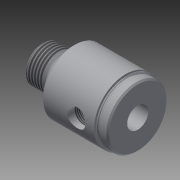
# Autodesk Inventor part: 12R000-0_rod_guide
Saved by Autodesk Inventor 2014 SP2 (Build 180246200, 246)
## iProperties
Created: 2019-01-29
Part Number: 12R000-0_rod_guide
Material: Generic
Catalog Web Link: www.cadenas.de
Description: Rod Guide-Original Line - Standard Air Cylinders
Vendor: BIMBA
Document SubType Name: Modeling
Designer: psadmin
Manufacturer: BIMBA
Mass: 28.8559 g
Surface Area: 85.2183 cm^2
Volume: 28.8559 cm^3
Density: 1 g/cm^3
Appearance: PSOLRGB-211-211-211
Category: PARTsolutions
Company: BIMBA
Title: 12R000-0_rod_guide
Author: Cadenas PARTsolutions
Comments: Original Line - Standard Air Cylinders
PSOL_IDENT_0: {$CADENAS_DATA\23d-libs\bimba\bimba\bimba_imperial\bimba_full_line\original_line_cylinders\standard_
PSOL_IDENT_1: air_cylinders\rod_guide.prj},251 {VTYP=3D},{NB=12R000-0_rod_guide},{LINA=12R000-0_rod_guide},{NN=Rod
PSOL_IDENT_2: Guide},{DATE=21.03.2018 14:31:21},{GEOMDATE=09.11.2017 12:44:00},{VERSION=},{LINEID=70},{WBVAR=MNT,
PSOL_IDENT_3: ACTING,NR,K,Q,T1,T2,T3,T4,MB,TRIM,CUSH,RODTRANS},{WBNUMERIC=MB,TRIM,CUSH,RODTRANS}  {NB=12R000-0_rod
PSOL_IDENT_4: _guide},{LINA=12R000-0_rod_guide},{KT=DUMMY},{PN=12R000},{BORE=1.25000000},{BOREPN=12},{MNT=},{MNTAL
PSOL_IDENT_5: G='' , 'Front Nose'},{ACTING=R},{ACTINGALG= '' , 'Single Acting' , 'R' , 'Reverse/Double Acting' },{
PSOL_IDENT_6: NR=},{NRALG= '' , 'N/A' },{K=},{Q=},{QALG= '' , 'Without Side Ported Rear Head' , 'Q' , 'With Side P
PSOL_IDENT_7: orted Rear Head' },{T1=},{T2=},{T3=},{T4=},{MB=0},{A1=2.0000},{A1N=1.5620},{A1P=2.0000},{A1B=0.0000}
PSOL_IDENT_8: ,{A2=0.6240},{A2N=0.6240},{A2P=0.6240},{A3=1.1250},{A3N=0.3110},{A3P=1.1250},{A4=0.2525},{A4N=0.6280
PSOL_IDENT_9: },{A4P=0.2525},{A5=0.0400},{A6=0.0000},{A6N=0.3750},{A6P=0.0000},{A7=0.4000},{A7N=0.9140},{A7P=0.400
PSOL_IDENT_10: 0},{A8=0.0300},{A8N=0.0300},{A8NR=0.0300},{D1=1.3265},{D1N=1.3265},{D1P=1.3265},{D1B=0.0000},{D2=1.2
PSOL_IDENT_11: 615},{D3=0.0000},{D3N=0.8120},{D3P=0.0000},{D4=0.8750},{D4N=0.4730},{D4P=0.8750},{D4NR=0.4395},{D5=0
PSOL_IDENT_12: .4420},{D5N=0.4420},{D5NR=0.4395},{C1=0.060},{C2=0.0300},{C2N=0.0600},{C2P=0.0300},{C3=0.0000},{C3N=
PSOL_IDENT_13: 0.0000},{C3P=0.0000},{C4=0.0600},{C4N=0.0600},{C4P=0.0600},{NDM=0.7500},{NDMN=0.7500},{NDMP=0.7500},
PSOL_IDENT_14: {TAB=UNF},{D6=0.7475},{D6N=0.7475},{D6P=0.7475},{A9=0.0940},{A9N=0.0940},{A9P=0.0940},{D7=0.6535},{D
PSOL_IDENT_15: 7N=0.6535},{D7P=0.6535},{A10=0.0965},{A10N=0.0965},{A10P=0.0965},{R1=0.0400},{R1N=0.0400},{R1P=0.040
PSOL_IDENT_16: 0},{D8=0.8750},{D9=0.7500},{D10=0.6880},{A11=0.9490},{A12=1.0740},{A13=1.2400},{A14=0.6250},{A14N=0.
PSOL_IDENT_17: 6250},{A14B=0.0000},{D11=0.2500},{D11N=0.2500},{NDM2=0.4050},{NDM2N=0.4050},{NDM2DP=0.3750},{THREAD=
PSOL_IDENT_18: 0},{HEX=0.4375},{HEXN=0.4375},{S1=0.0000},{B1=0.0000},{B2=0.0000},{B22=0.0000},{DB=0.0000},{B3=0.000
PSOL_IDENT_19: 0},{B4=0.0000},{X1=0.0000},{X2=0.0000},{NDM3=0.0000},{NDM4=0.0000},{NDM4DP=0.0000},{DD=0.0000},{CB=0
PSOL_IDENT_20: .0000},{CBDP=0.0000},{PORT=1},{XT=0.0000},{XTX=0.0000},{XT1=0.0000},{XT2=0.0000},{NDMH=0.0000},{OD=1
PSOL_IDENT_21: .3265},{ID=1.2615},{G=0.0000},{PNUT=0.5300},{TRIM=0},{C11=0.0000},{C22=0.0000},{C33=0.0000},{C44=0.0
PSOL_IDENT_22: 000},{C55=0.0000},{CD1=0.0000},{CD2=0.0000},{CD3=0.0000},{CNDM3=0.0000},{CTAB3=0.0000},{CUSH=0},{XX=
PSOL_IDENT_23: 0.00000},{LCD=0.0000},{RODTRANS=0.00000}
NN: Rod Guide
NT: Original Line - Standard Air Cylinders
NB: 12R000-0_rod_guide
NBSYN: $PN.-$RODTRANS._rod_guide
LINA: 12R000-0_rod_guide
BORE: 0
BOREPN: 12
MNT: Front Nose
MNTALG: '' , 'Front Nose'
ACTING: Reverse/Double Acting
NR: N/A
K: Standard
Q: Without Side Ported Rear Head
T1: without T1
T2: without T2
T3: without T3
T4: without T4
MB: 0
A1N: 1.562
A1P: 2
A1B: 0
A2N: 0.624
A2P: 0.624
A3N: 0.311
A3P: 1.125
A4N: 0.628
A4P: 0.2525
A5: 0.04
A6N: 0.375
A6P: 0
A7N: 0.914
A7P: 0.4
A8N: 0.03
A8NR: 0.03
D1N: 1.3265
D1P: 1.3265
D1B: 0
D2: 1.2615
D3N: 0.812
D3P: 0
D4N: 0.473
D4P: 0.875
D4NR: 0.4395
D5N: 0.442
D5NR: 0.4395
C1: 0.06
C2N: 0.06
C2P: 0.03
C3N: 0
C3P: 0
C4N: 0.06
C4P: 0.06
NDMN: 0.75
NDMP: 0.75
TAB: UNF
D6N: 0.7475
D6P: 0.7475
A9N: 0.094
A9P: 0.094
D7N: 0.6535
D7P: 0.6535
A10N: 0.0965
A10P: 0.0965
R1N: 0.04
R1P: 0.04
D8: 0.875
D9: 0.75
D10: 0.688
A11: 0.949
A12: 1.074
A13: 1.24
A14N: 0.625
A14B: 0
D11N: 0.25
NDM2N: 0.405
NDM2DP: 0.375
HEXN: 0.4375
S1: 0
B1: 0
B2: 0
B22: 0
DB: 0
B3: 0
B4: 0
X1: 0
X2: 0
NDM3: 0
NDM4: 0
NDM4DP: 0
DD: 0
CB: 0
CBDP: 0
XTX: 0
XT1: 0
XT2: 0
NDMH: 0
TRIM: 0
C11: 0
C22: 0
C33: 0
C44: 0
C55: 0
CD1: 0
CD2: 0
CD3: 0
CNDM3: 0
CTAB3: 0.0000
CUSH: 0
LCD: 0
RODTRANS: 0
SUPPLIER: BIMBA
ARTICLENO: 12R000-0_rod_guide
BOMINFO: 12R000-0_rod_guide
CREATOR: CADENAS GmbH
Autodesk Inventor part; units mm, degrees
sketch "Sketch_2" plane through (0, 0, 0) normal (0, 0, 1) x (1, 0, 0)
  line L0 (15.8496, 0) -> (0, 0)
  line L1 (0, 0) -> (0, 8.589)
  line L2 (0, 8.589) -> (0.936, 9.525)
  line L3 (0.936, 9.525) -> (9.3565, 9.525)
  line L4 (9.3565, 9.525) -> (10.2956, 8.594)
  arc A0 (10.2956, 8.594) -> (11.0109, 8.2995) centre (11.0109, 9.3154) ccw
  line L5 (11.0109, 8.2995) -> (12.446, 8.2995)
  arc A1 (12.446, 8.2995) -> (13.462, 9.3155) centre (12.446, 9.3154) ccw
  line L6 (13.462, 9.3155) -> (13.462, 9.4932)
  line L7 (13.462, 9.4932) -> (15.8496, 9.4932)
  line L8 (15.8496, 9.4932) -> (15.8496, 0)
  line L9 (15.8496, 0) -> (0, 0)
  constraints: 20 end point, 4 point on circle, 2 centre point
revolve "Revolution1" add sketch "Sketch_2" angle 360 about axis through (15.8496, 0, 0) along (1, 0, 0)
thread "Thread1" size "3/4-16 UNF" class "2A" standard "ANSI Unified Screw Threads" full length
sketch "Sketch_3" plane through (0, 0, 0) normal (0, 0, 1) x (1, 0, 0)
  line L0 (50.8, 0) -> (15.8496, 0)
  line L1 (15.8496, 0) -> (15.8496, 15.3226)
  line L2 (15.8496, 15.3226) -> (17.3736, 16.8466)
  line L3 (17.3736, 16.8466) -> (44.3865, 16.8466)
  line L4 (44.3865, 16.8466) -> (44.3865, 15.0051)
  line L5 (44.3865, 15.0051) -> (45.4025, 15.0051)
  line L6 (45.4025, 15.0051) -> (46.4185, 16.021)
  line L7 (46.4185, 16.021) -> (50.038, 16.021)
  line L8 (50.038, 16.021) -> (50.8, 15.2591)
  line L9 (50.8, 15.2591) -> (50.8, 0)
  line L10 (50.8, 0) -> (15.8496, 0)
  constraints: 22 end point
revolve "Revolution2" add sketch "Sketch_3" angle 360 about axis through (50.8, 0, 0) along (1, 0, 0)
sketch "Sketch3" plane through (0, 0, 0) normal (-1, 0, 0) x (0, 0, 1)
  point P0 (0, 0)
hole "Hole1" at (0, 0, 0) direction (1, 0, 0) diameter 11.2268 depth 50.8 countersink diameter 12.7508 countersink angle 90
sketch "Sketch_40" plane through (0, 0, 0) normal (0, 1, 0) x (-1, 0, 0)
  line L0 (-34.925, 16.8466) -> (-34.925, 0)
  line L1 (-34.925, 0) -> (-38.1, 0)
  line L2 (-38.1, 0) -> (-38.1, 5.9544)
  line L3 (-38.1, 5.9544) -> (-39.4671, 7.3216)
  line L4 (-39.4671, 7.3216) -> (-39.7645, 16.8466)
  line L5 (-39.7645, 16.8466) -> (-34.925, 16.8466)
  line L6 (-34.925, 16.8466) -> (-34.925, 0)
  constraints: 14 end point
revolve "Revolution3" cut sketch "Sketch_40" angle 360 about axis through (34.925, 0, 16.8466) along (0, 0, 1)
thread "Thread2" size "1/8" designation "1/8 - 27 NPT" standard "NPT" length 5.7178
sketch "Sketch_47" plane through (0, 0, 0) normal (0, 0, 1) x (1, 0, 0)
  line L0 (45.4025, 0) -> (44.3865, 0)
  line L1 (44.3865, 15.7133) -> (44.3865, 14.7511)
  line L2 (44.3865, 14.7511) -> (45.4025, 14.7511)
  line L3 (45.4025, 14.7511) -> (45.4025, 15.0051)
  line L4 (45.4025, 15.0051) -> (44.8945, 15.0051)
  line L5 (44.8945, 15.0051) -> (44.5199, 15.3797)
  arc A0 (44.5199, 15.5593) -> (44.5199, 15.3797) centre (44.6097, 15.4695) ccw
  line L6 (44.5199, 15.5593) -> (45.723, 16.7624)
  line L7 (45.723, 16.7624) -> (45.723, 16.8466)
  line L8 (45.723, 16.8466) -> (45.5198, 16.8466)
  line L9 (45.5198, 16.8466) -> (44.3865, 15.7133)
  constraints: 20 end point, 2 point on circle, 1 centre point
revolve "Revolution4" add sketch "Sketch_47" angle 360 about axis through (45.4025, 0, 0) along (1, 0, 0)
ref_plane "dp1_XY" through (15.8496, 9.4932, 0) normal (0, 0, 1) x (1, 0, 0)
ref_plane "dp1_YZ" through (15.8496, 9.4932, 0) normal (1, 0, 0) x (0, 1, 0)
ref_plane "dp1_ZX" through (15.8496, 9.4932, 0) normal (0, 1, 0) x (0, 0, 1)
ref_plane "dp2_XY" through (15.8496, -9.4932, 0) normal (0, 0, 1) x (1, 0, 0)
ref_plane "dp2_YZ" through (15.8496, -9.4932, 0) normal (1, 0, 0) x (0, 1, 0)
ref_plane "dp2_ZX" through (15.8496, -9.4932, 0) normal (0, 1, 0) x (0, 0, 1)
ref_plane "hh_XY" through (0, 9.525, 0) normal (0, 0, 1) x (1, 0, 0)
ref_plane "hh_YZ" through (0, 9.525, 0) normal (1, 0, 0) x (0, 1, 0)
ref_plane "hh_ZX" through (0, 9.525, 0) normal (0, 1, 0) x (0, 0, 1)
ref_plane "port_XY" through (34.925, 0, 0) normal (0, 0, 1) x (1, 0, 0)
ref_plane "port_YZ" through (34.925, 0, 0) normal (1, 0, 0) x (0, 1, 0)
ref_plane "port_ZX" through (34.925, 0, 0) normal (0, 1, 0) x (0, 0, 1)
ref_plane "rod_guide_XY" through (0, 0, 0) normal (1, 0, 0) x (0, 0, -1)
ref_plane "rod_guide_YZ" through (0, 0, 0) normal (0, 0, -1) x (0, 1, 0)
ref_plane "rod_guide_ZX" through (0, 0, 0) normal (0, 1, 0) x (1, 0, 0)
ref_plane "s1_XY" through (13.462, 0, 0) normal (0, 0, 1) x (1, 0, 0)
ref_plane "s1_YZ" through (13.462, 0, 0) normal (1, 0, 0) x (0, 1, 0)
ref_plane "s1_ZX" through (13.462, 0, 0) normal (0, 1, 0) x (0, 0, 1)
ref_plane "s2_XY" through (15.8496, 0, 0) normal (0, 0, 1) x (1, 0, 0)
ref_plane "s2_YZ" through (15.8496, 0, 0) normal (1, 0, 0) x (0, 1, 0)
ref_plane "s2_ZX" through (15.8496, 0, 0) normal (0, 1, 0) x (0, 0, 1)
ref_plane "t1_XY" through (15.8496, 0, 0) normal (1, 0, 0) x (0, 0, -1)
ref_plane "t1_YZ" through (15.8496, 0, 0) normal (0, 0, -1) x (0, 1, 0)
ref_plane "t1_ZX" through (15.8496, 0, 0) normal (0, 1, 0) x (1, 0, 0)
ref_plane "t111_XY" through (15.8496, 0, 0) normal (1, 0, 0) x (0, 0, -1)
ref_plane "t111_YZ" through (15.8496, 0, 0) normal (0, 0, -1) x (0, 1, 0)
ref_plane "t111_ZX" through (15.8496, 0, 0) normal (0, 1, 0) x (1, 0, 0)
ref_plane "to_foot_bracket_XY" through (15.8496, 0, 0) normal (1, 0, 0) x (0, 0, -1)
ref_plane "to_foot_bracket_YZ" through (15.8496, 0, 0) normal (0, 0, -1) x (0, 1, 0)
ref_plane "to_foot_bracket_ZX" through (15.8496, 0, 0) normal (0, 1, 0) x (1, 0, 0)
ref_plane "to_nut_XY" through (13.462, 0, 0) normal (1, 0, 0) x (0, 0, -1)
ref_plane "to_nut_YZ" through (13.462, 0, 0) normal (0, 0, -1) x (0, 1, 0)
ref_plane "to_nut_ZX" through (13.462, 0, 0) normal (0, 1, 0) x (1, 0, 0)
ref_plane "to_rod_XY" through (0, 0, 0) normal (1, 0, 0) x (0, 0, -1)
ref_plane "to_rod_YZ" through (0, 0, 0) normal (0, 0, -1) x (0, 1, 0)
ref_plane "to_rod_ZX" through (0, 0, 0) normal (0, 1, 0) x (1, 0, 0)
ref_plane "to_screw_XY" through (34.925, 0, 0) normal (0, 1, 0) x (1, 0, 0)
ref_plane "to_screw_YZ" through (34.925, 0, 0) normal (1, 0, 0) x (0, 0, -1)
ref_plane "to_screw_ZX" through (34.925, 0, 0) normal (0, 0, -1) x (0, 1, 0)
ref_plane "to_trunnion_brackets_XY" through (0, 0, 0) normal (0, 1, 0) x (1, 0, 0)
ref_plane "to_trunnion_brackets_YZ" through (0, 0, 0) normal (1, 0, 0) x (0, 0, -1)
ref_plane "to_trunnion_brackets_ZX" through (0, 0, 0) normal (0, 0, -1) x (0, 1, 0)
ref_plane "to_trunnion_brackets1_XY" through (0, 0, 0) normal (0, 1, 0) x (1, 0, 0)
ref_plane "to_trunnion_brackets1_YZ" through (0, 0, 0) normal (1, 0, 0) x (0, 0, -1)
ref_plane "to_trunnion_brackets1_ZX" through (0, 0, 0) normal (0, 0, -1) x (0, 1, 0)
ref_plane "to_trunnion_brackets2_XY" through (0, 0, 0) normal (0, 1, 0) x (1, 0, 0)
ref_plane "to_trunnion_brackets2_YZ" through (0, 0, 0) normal (1, 0, 0) x (0, 0, -1)
ref_plane "to_trunnion_brackets2_ZX" through (0, 0, 0) normal (0, 0, -1) x (0, 1, 0)
ref_plane "to_tube_XY" through (45.4025, 0, 0) normal (1, 0, 0) x (0, 0, -1)
ref_plane "to_tube_YZ" through (45.4025, 0, 0) normal (0, 0, -1) x (0, 1, 0)
ref_plane "to_tube_ZX" through (45.4025, 0, 0) normal (0, 1, 0) x (1, 0, 0)
body "Solid1"
